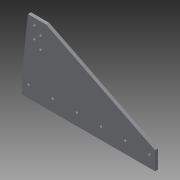
# Autodesk Inventor part: rail mounting bracket
Saved by Autodesk Inventor 2015 SP1 (Build 190203100, 203)
## iProperties
Created: 2015-01-15
Part Number: rail mounting bracket
Material: Generic
Document SubType Name: Modeling
Designer: Jarod
Density: 1 g/cm^3
Appearance: Default
Author: Jarod
Autodesk Inventor part; units mm, degrees
ref_plane "YZ Plane" through (0, 0, 0) normal (1, 0, 0) x (0, 1, 0)
ref_plane "XZ Plane" through (0, 0, 0) normal (0, 1, 0) x (-1, 0, 0)
ref_plane "XY Plane" through (0, 0, 0) normal (0, 0, 1) x (1, 0, 0)
sketch "Sketch1" plane through (0, 0, 0) normal (0, 0, 1) x (1, 0, 0)
  line L0 (0, 0) -> (279.4, 0) construction
  line L1 (279.4, 0) -> (279.4, 152.4) construction
  line L2 (279.4, 152.4) -> (0, 152.4) construction
  line L3 (0, 152.4) -> (0, 0) construction
  line L4 (0, 0) -> (279.4, 0)
  line L5 (0, 0) -> (0, 38.1)
  line L6 (0, 0) -> (38.1, 0) construction
  line L7 (279.4, 0) -> (279.4, 38.1)
  line L8 (279.4, 0) -> (317.5, 0) construction
  line L9 (279.4, 152.4) -> (57.15, 152.4) construction
  line L10 (279.4, 152.4) -> (501.65, 152.4) construction
  line L11 (57.15, 152.4) -> (19.05, 152.4) construction
  line L12 (0, 38.1) -> (19.05, 152.4)
  line L13 (19.05, 152.4) -> (57.15, 152.4)
  line L14 (57.15, 152.4) -> (279.4, 38.1)
  circle A0 centre (12.7, 25.4) radius 3.175
  circle A1 centre (63.5, 25.4) radius 3.175
  circle A2 centre (215.9, 25.4) radius 3.175
  circle A3 centre (266.7, 25.4) radius 3.175
  circle A4 centre (31.75, 139.7) radius 3.175
  circle A5 centre (44.45, 127) radius 3.175
  circle A6 centre (31.75, 114.3) radius 3.175
  circle A7 centre (44.45, 101.6) radius 3.175
  circle A8 centre (114.3, 25.4) radius 3.175
  circle A9 centre (165.1, 25.4) radius 3.175
  dimension "d0" = 279.4
  dimension "d1" = 152.4
  dimension "d2" = 12.7
  dimension "d3" = 50.8
  dimension "d4" = 50.8
  dimension "d5" = 12.7
  dimension "d6" = 25.4
  dimension "d7" = 25.4
  dimension "d8" = 25.4
  dimension "d9" = 25.4
  dimension "d10" = 38.1
  dimension "d11" = 90
  dimension "d12" = 38.1
  dimension "d13" = 90
  dimension "d14" = 222.25
  dimension "d15" = 180
  dimension "d16" = 38.1
  dimension "d17" = 12.7
  dimension "d18" = 12.7
  dimension "d19" = 12.7
  dimension "d20" = 12.7
  dimension "d21" = 12.7
  dimension "d22" = 25.4
  dimension "d23" = 38.1
  dimension "d24" = 50.8
  dimension "d25" = 6.35
  dimension "d26" = 6.35
  dimension "d27" = 6.35
  dimension "d28" = 6.35
  dimension "d29" = 6.35
  dimension "d30" = 6.35
  dimension "d31" = 6.35
  dimension "d32" = 6.35
  dimension "d35" = 50.8
  dimension "d36" = 50.8
  dimension "d37" = 50.8
  dimension "d38" = 6.35
  dimension "d39" = 6.35
  constraints: 30 end point, 10 centre point, 10 coincident, 6 horizontal, 3 collinear, 3 equal length, 2 parallel, 1 perpendicular, 1 point on line
  measures "d0" distance of L2.end L1.end
  measures "d1" distance of L1.end L0.end
  measures "d2" distance from line of point (12.7, 25.4) L3
  measures "d3" distance of point (63.5, 25.4) point (12.7, 25.4)
  measures "d4" distance of point (266.7, 25.4) point (215.9, 25.4)
  measures "d5" distance from line of L1 point (266.7, 25.4)
  measures "d6" distance from line of L0 point (266.7, 25.4)
  measures "d7" distance from line of L0 point (215.9, 25.4)
  measures "d8" distance from line of L0 point (63.5, 25.4)
  measures "d9" distance from line of L0 point (12.7, 25.4)
  measures "d10" distance of L0.start L5.end
  measures "d11" angle of L6 L5
  measures "d12" distance of L0.end L7.end
  measures "d13" angle of L8 L7
  measures "d14" distance of L1.end L9.end
  measures "d15" angle of L9 L10
  measures "d16" distance of L9.end L11.end
  measures "d17" horizontal distance of point (31.75, 139.7) L11.end
  measures "d18" horizontal distance of point (44.45, 127) L9.end
  measures "d19" horizontal distance of L11.end point (31.75, 114.3)
  measures "d20" horizontal distance of L9.end point (44.45, 101.6)
  measures "d21" distance from line of L11 point (31.75, 139.7)
  measures "d22" distance from line of L2 point (44.45, 127)
  measures "d23" distance from line of L11 point (31.75, 114.3)
  measures "d24" distance from line of point (44.45, 101.6) L11
  measures "d25" diameter of A0
  measures "d26" diameter of A1
  measures "d27" diameter of A2
  measures "d28" diameter of A3
  measures "d29" diameter of A4
  measures "d30" diameter of A5
  measures "d31" diameter of A6
  measures "d32" diameter of A7
  measures "d35" distance of point (114.3, 25.4) point (63.5, 25.4)
  measures "d36" distance of point (165.1, 25.4) point (114.3, 25.4)
  measures "d37" distance of point (215.9, 25.4) point (165.1, 25.4)
  measures "d38" diameter of A8
  measures "d39" diameter of A9
extrude "Extrusion2" add sketch "Sketch1" along normal blind 6.35
body "Solid2"
